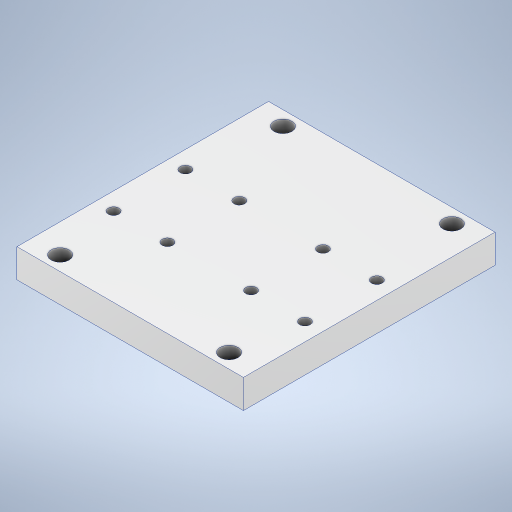
# Autodesk Inventor part: Lateral da caixa de sustentação
Saved by Autodesk Inventor 2023 (Build 270158000, 158)
## iProperties
Created: 2023-04-29
Part Number: Lateral da caixa de sustentação
Material: Aluminum 6061
Document SubType Name: Sheet Metal
Designer: Mateus PC
Density: 2.7 g/cm^3
Sheet Metal Rule: Default_mm
Appearance: Aluminum - Flat
Author: Mateus PC
Autodesk Inventor part; units mm, degrees
ref_plane "YZ Plane" through (0, 0, 0) normal (1, 0, 0) x (0, 1, 0)
ref_plane "XZ Plane" through (0, 0, 0) normal (0, 1, 0) x (-1, 0, 0)
ref_plane "XY Plane" through (0, 0, 0) normal (0, 0, 1) x (1, 0, 0)
sketch "Sketch1" plane through (0, 0, 0) normal (0, 1, 0) x (-1, 0, 0)
  line L0 (0, 0) -> (63, 0)
  line L1 (63, 0) -> (63, -70)
  line L2 (63, -70) -> (0, -70)
  line L3 (0, -70) -> (0, 0)
  dimension "d0" = 70
  dimension "d1" = 63
  constraints: 8 end point, 2 parallel, 1 horizontal, 1 perpendicular
  measures "d0" distance of L0.end L1.end
  measures "d1" distance of L1.end L2.end
extrude "Extrusion1" add sketch "Sketch1" along normal blind 8
sketch "Sketch2" plane through (0, 8, 0) normal (0, 1, 0) x (1, 0, 0)
  line L0 (0, 70) -> (-63, 70) projected
  line L1 (-63, 70) -> (-63, 0) projected
  line L2 (0, 0) -> (0, 70) projected
  point P0 (-58.125, 42)
  point P1 (-43.125, 42)
  point P2 (-58.125, 22)
  point P3 (-43.125, 22)
  point P4 (-19.875, 42)
  point P5 (-19.875, 22)
  point P6 (-4.875, 42)
  point P7 (-4.875, 22)
  dimension "d4" = 70
  dimension "d5" = 63
  dimension "d8" = 15
  dimension "d11" = 20
  dimension "d18" = 20
  dimension "d21" = 15
  dimension "d24" = 23.25
  dimension "d25" = 0
  dimension "d26" = 28
  dimension "d27" = 53.25
  dimension "d28" = -4.875
  constraints: 2 horizontal, 2 vertical, 6 other
  measures "d4" distance of L0.end L1.end
  measures "d5" distance of L0.start L0.end
  measures "d8" distance of point (-58.125, 42) point (-43.125, 42)
  measures "d11" distance of point (-58.125, 42) point (-58.125, 22)
  measures "d18" distance of point (-19.875, 42) point (-19.875, 22)
  measures "d21" distance of point (-19.875, 42) point (-4.875, 42)
  measures "d24" distance of point (-43.125, 42) point (-19.875, 42)
  measures "d25" vertical distance of point (-43.125, 42) point (-19.875, 42)
  measures "d26" distance from line of point (-43.125, 42) L0
  measures "d27" distance of point (-58.125, 42) point (-4.875, 42)
  measures "d28" distance from line of L2 point (-4.875, 42)
hole "Hole1" at (-58.125, 8, -42) at (-43.125, 8, -42) at (-58.125, 8, -22) at (-43.125, 8, -22) at (-19.875, 8, -42) at (-19.875, 8, -22) at (-4.875, 8, -42) at (-4.875, 8, -22) direction (0, -1, 0) diameter 3 end through all
sketch "Sketch3" plane through (0, 8, 0) normal (0, 1, 0) x (1, 0, 0)
  line L0 (0, 0) -> (0, 70) projected
  line L1 (-63, 0) -> (0, 0) projected
  point P0 (-8, 4)
  point P1 (-55, 4)
  point P2 (-8, 66)
  point P3 (-55, 66)
  dimension "d38" = 47
  dimension "d41" = 62
  dimension "d44" = 63
  dimension "d45" = 70
  dimension "d46" = 4
  dimension "d47" = 8
  constraints: 1 horizontal, 1 vertical, 3 other
  measures "d38" distance of point (-8, 4) point (-55, 4)
  measures "d41" distance of point (-8, 4) point (-8, 66)
  measures "d44" distance of L1.start L0.start
  measures "d45" distance of L0.start L0.end
  measures "d46" distance from line of L1 point (-8, 4)
  measures "d47" distance from line of L0 point (-8, 4)
hole "Hole2" at (-8, 8, -4) at (-55, 8, -4) at (-8, 8, -66) at (-55, 8, -66) direction (0, -1, 0) diameter 5 end through all
equation "\"d28\" = 0.5 * d27 - 0.5 * d5"
equation "\"d34\" = Thickness"
equation "\"d46\" = 0.5 * d45 - 0.5 * d41"
equation "\"d47\" = 0.5 * d44 - 0.5 * d38"
equation "\"d53\" = Thickness"
equation "\"BendRadius\" = Thickness"
equation "\"BendReliefWidth\" = Thickness"
equation "\"BendReliefDepth\" = 0.5 * Thickness"
equation "\"CornerReliefSize\" = 4 * Thickness"
equation "\"MinimumRemnant\" = 2 * Thickness"
equation "\"TransitionRadius\" = BendRadius"
equation "\"JacobiRadiusSize\" = BendRadius"
equation "\"GapSize\" = Thickness"
equation "\"Thickness\" = 0.5"
body "Solid1"
